Autodesk Inventor part; units mm, degrees
(part 3 of 3)
  line L422 (119.3772, -52.824) -> (120.0796, -50.6806) construction
  line L423 (120.0796, -50.6806) -> (122.6545, -48.1402) construction
  spline S98 degree 3 poles (122.6545, -48.1402) (125.227, -45.6023) (125.3462, -39.3878) (125.4242, -37.8716) knots 0.931034 0.931034 0.931034 0.931034 0.948276 0.948276 0.948276 0.948276
  line L424 (122.6545, -48.1402) -> (125.227, -45.6023) construction
  line L425 (125.227, -45.6023) -> (125.3462, -39.3878) construction
  line L426 (125.3462, -39.3878) -> (125.4242, -37.8716) construction
  spline S99 degree 3 poles (125.4242, -37.8716) (125.5236, -37.2768) (125.9505, -34.7145) (126.0454, -34.112) knots 0.948276 0.948276 0.948276 0.948276 0.965517 0.965517 0.965517 0.965517
  line L427 (125.4242, -37.8716) -> (125.5236, -37.2768) construction
  line L428 (125.5236, -37.2768) -> (125.9505, -34.7145) construction
  line L429 (125.9505, -34.7145) -> (126.0454, -34.112) construction
  spline S100 degree 3 poles (126.0454, -34.112) (126.1537, -33.429) (126.6324, -32.5563) (126.9372, -32.0652) knots 0.965517 0.965517 0.965517 0.965517 0.982759 0.982759 0.982759 0.982759
  line L430 (126.0454, -34.112) -> (126.1537, -33.429) construction
  line L431 (126.1537, -33.429) -> (126.6324, -32.5563) construction
  line L432 (126.6324, -32.5563) -> (126.9372, -32.0652) construction
  spline S101 degree 3 poles (126.9372, -32.0652) (127.2424, -31.5748) (127.1429, -31.1233) (127.3225, -30.7663) knots 0.982759 0.982759 0.982759 0.982759 1 1 1 1
  line L433 (126.9372, -32.0652) -> (127.2424, -31.5748) construction
  line L434 (127.2424, -31.5748) -> (127.1429, -31.1233) construction
  line L435 (127.1429, -31.1233) -> (127.3225, -30.7663) construction
  constraints: 116 end point, 303 other
extrude "Wyciągnięcie proste9" cut sketch "Szkic13" against normal blind 2
sketch "Szkic17" plane through (0, 0, 8.64) normal (0, 0, 1) x (1, 0, 0)
  circle A0 centre (-81.484, -2.25) radius 1.5
  line L0 (-60.1, -49) -> (-76.3, -49) projected
  circle A1 centre (-6.484, -2.25) radius 1.5
  circle A2 centre (68.516, -2.25) radius 1.5
  circle A3 centre (-81.484, 41.75) radius 1.5
  circle A4 centre (-6.484, 41.75) radius 1.5
  circle A5 centre (68.516, 41.75) radius 1.5
  line L1 (-1.3, -49) -> (3.2327, -49) projected
  line L2 (73.7, -49) -> (78.2327, -49) projected
  point P0 (0, 0)
  dimension "d137" = 3
  dimension "d138" = 5.184
  dimension "d139" = 46.75
  dimension "d140" = 3
  dimension "d141" = 3
  dimension "d142" = 75
  dimension "d143" = 75
  dimension "d144" = 3
  dimension "d145" = 44
  dimension "d146" = 3
  dimension "d147" = 44
  dimension "d148" = 3
  dimension "d149" = 44
  dimension "d157" = 46.75
  dimension "d158" = 46.75
  constraints: 6 centre point
  measures "d137" diameter of A0
  measures "d138" horizontal distance of A0.centre L0.end
  measures "d139" vertical distance of A0.centre L0.end
  measures "d140" diameter of A1
  measures "d141" diameter of A2
  measures "d142" distance of A1.centre A0.centre
  measures "d143" distance of A2.centre A1.centre
  measures "d144" diameter of A3
  measures "d145" distance of A3.centre A0.centre
  measures "d146" diameter of A4
  measures "d147" distance of A4.centre A1.centre
  measures "d148" diameter of A5
  measures "d149" distance of A5.centre A2.centre
  measures "d157" distance from line of L1 A1.centre
  measures "d158" distance from line of A2.centre L2
ref_plane "Płaszczyzna konstrukcyjna11" through (-85.1, 41.2, 8.64) normal (-1, 0, 0) x (0, 0, 1)
sketch "Szkic18" plane through (-85.1, 41.2, 8.64) normal (-1, 0, 0) x (0, 0, 1)
  line L0 (0, 7.8) -> (17.7931, 7.8) construction
  line L1 (0, 7.8) -> (0, 0) projected
  line L2 (0, 7.8) -> (32.4855, 7.8) construction
  line L3 (105.01, 0) -> (0, 0) projected
  line L4 (105.01, 0) -> (0, 0) projected
  line L5 (105.01, 7.8) -> (105.01, 0) projected
  line L6 (95.01, 0) -> (87.21, 7.8)
  line L7 (105.01, 0) -> (118.7125, 0) construction
  line L8 (105.01, 7.8) -> (0, 7.8) projected
  line L9 (87.21, 7.8) -> (0, 7.8)
  line L10 (0, 7.8) -> (0, 0)
  line L11 (0, 0) -> (95.01, 0)
  line L12 (101.1463, -91.4) -> (2.96, -91.4) projected
  line L13 (95.01, 0) -> (188.9531, 0) construction
  line L14 (105.01, -82.4) -> (0, -82.4) projected
  line L15 (105.01, -82.4) -> (105.01, -90.2) projected
  line L16 (95.01, -82.4) -> (87.21, -90.2)
  line L17 (95.01, -82.4) -> (116.6917, -82.4) construction
  line L18 (0, -90.2) -> (0, -82.4) projected
  line L19 (95.01, -82.4) -> (0, -82.4)
  line L20 (0, -82.4) -> (0, -90.2)
  line L21 (101.1463, -90.2) -> (2.96, -90.2) projected
  line L22 (87.21, -90.2) -> (0, -90.2)
  point P0 (-8.64, -41.2)
  dimension "d175" = 10
  dimension "d176" = 135
  dimension "d178" = 10
  dimension "d179" = 135
  constraints: 26 end point, 7 horizontal, 4 point on line, 2 perpendicular, 1 collinear
  measures "d175" distance from line of L6.start L5
  measures "d176" angle of L7 L6
  measures "d178" distance from line of L15 L16.start
  measures "d179" angle of L16 L17
extrude "Wyciągnięcie proste11" cut sketch "Szkic18" against normal blind 184 contours L8 L6 L3 L1 | L16 L21 L22 L18 L14
extrude "Wyciągnięcie proste12" cut sketch "Szkic17" against normal blind 5
ref_plane "Płaszczyzna konstrukcyjna12" through (-100, -50.2, 115.25) normal (1, 0, 0) x (0, 0, -1)
sketch "Szkic19" plane through (-100, -50.2, 115.25) normal (1, 0, 0) x (0, 0, -1)
  line L0 (106.61, 1.2) -> (106.61, 99.2) projected
  line L1 (106.61, 43.2) -> (103.61, 43.2)
  line L2 (103.61, 43.2) -> (103.61, 96.2)
  line L3 (103.61, 96.2) -> (106.61, 96.2)
  line L4 (106.61, 96.2) -> (106.61, 43.2)
  point P0 (115.25, 50.2)
  point P1 (106.61, 1.2)
  point P2 (106.61, 99.2)
  dimension "d160" = 42
  dimension "d161" = 3
  dimension "d162" = 53
  constraints: 8 end point, 2 coincident, 2 parallel, 1 horizontal, 1 perpendicular, 1 point on line
  measures "d160" distance of L1.start L0.start
  measures "d161" distance of L2.end L3.end
  measures "d162" distance of L1.end L2.end
extrude "Wyciągnięcie proste13" cut sketch "Szkic19" against normal blind 2.5
chamfer "Faza3" distance 2 angle 45 1 edges at (-100, 19.5, 11.64)
sketch "Szkic20" plane through (0, 0, 115.25) normal (0, 0, 1) x (1, 0, 0)
  circle A0 centre (-80.7, 45.2) radius 1.5
  circle A1 centre (-80.7, 45.2) radius 1.5 projected
  circle A2 centre (-80.7, -45.2) radius 1.5
  circle A3 centre (-80.7, -45.2) radius 1.5 projected
  line L0 (-80.7, -45.2) -> (-117.5557, -45.2)
  line L1 (-80.7, -45.2) -> (127.3171, -45.2)
  line L2 (-80.7, 45.2) -> (115.4079, 45.2)
  line L3 (-80.7, 45.2) -> (-126.0914, 45.2)
  circle A4 centre (-105, 45.2) radius 1.5
  line L4 (-100, -50.2) -> (-100, 50.2) projected
  line L5 (-110, 55) -> (-110, -55) projected
  line L6 (-105, 0) -> (-106.6545, 0)
  line L7 (0, 34.4535) -> (0, 31.8021)
  circle A5 centre (-105, -45.2) radius 1.5
  circle A6 centre (105, 45.2) radius 1.5
  circle A7 centre (105, -45.2) radius 1.5
  point P0 (0, 0)
  dimension "d168" = 3
  dimension "d169" = 3
  dimension "d170" = 3
  dimension "d171" = 10
  dimension "d172" = 5
  constraints: 12 end point, 6 centre point, 5 horizontal, 3 symmetric about line, 2 concentric, 1 point on line, 1 vertical, 3 other
  measures "d168" diameter of A0
  measures "d169" diameter of A2
  measures "d170" diameter of A4
  measures "d171" distance between parallel lines of L4 L5
  measures "d172" distance from line of L5 A4.centre
extrude "Wyciągnięcie proste14" cut sketch "Szkic20" against normal blind 10 contours A7 L1 | L1 A7 | A6 L2 | L2 A6 | A4 L3 | L3 A4 | A5 L0 | L0 A5
equation "\"d36\" = 0.5 * d35"
equation "\"d44\" = 0.5 * d43"
equation "\"d59\" = d57"
